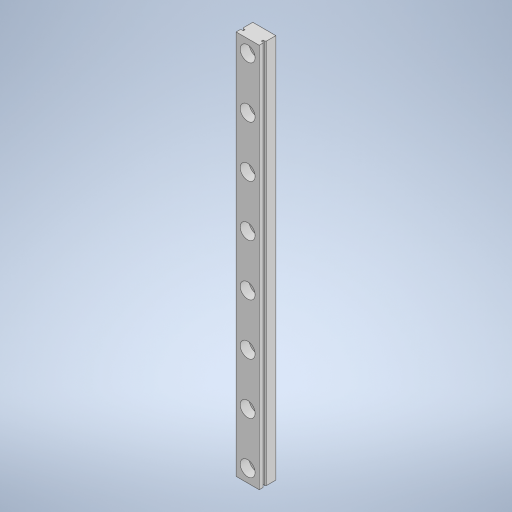
# Autodesk Inventor part: rail
Saved by Autodesk Inventor 2024 (Build 280153000, 153)
## iProperties
Created: 2025-06-01
Part Number: rail
Material: 一般
Document SubType Name: Modeling
Designer: 1412z
Density: 1 g/cm^3
Appearance: 既定
Author: 1412z
Autodesk Inventor part; units mm, degrees
ref_plane "YZ Plane" through (0, 0, 0) normal (1, 0, 0) x (0, 1, 0)
ref_plane "XZ Plane" through (0, 0, 0) normal (0, 1, 0) x (-1, 0, 0)
ref_plane "XY Plane" through (0, 0, 0) normal (0, 0, 1) x (1, 0, 0)
sketch "スケッチ1" plane through (0, 0, 0) normal (0, 0, 1) x (1, 0, 0)
  line L0 (-4.5, 75) -> (4.5, 75)
  line L1 (4.5, 75) -> (4.5, -75)
  line L2 (4.5, -75) -> (-4.5, -75)
  line L3 (-4.5, -75) -> (-4.5, 75)
  line L4 (-4.5, 75) -> (4.5, -75) construction
  line L5 (4.5, 75) -> (-4.5, -75) construction
  circle A0 centre (0, 70) radius 1.7
  circle A1 centre (0, 50) radius 1.7
  circle A2 centre (0, 30) radius 1.7
  circle A3 centre (0, 10) radius 1.7
  circle A4 centre (0, -10) radius 1.7
  circle A5 centre (0, -30) radius 1.7
  circle A6 centre (0, -50) radius 1.7
  circle A7 centre (0, -70) radius 1.7
  point P0 (0, 0)
  dimension "d0" = 9
  dimension "d1" = 150
  dimension "d2" = 3.4
  dimension "d3" = 3.4
  dimension "d4" = 3.4
  dimension "d5" = 3.4
  dimension "d6" = 3.4
  dimension "d7" = 3.4
  dimension "d8" = 3.4
  dimension "d9" = 3.4
  constraints: 12 end point, 8 centre point, 2 midpoint, 2 parallel, 1 horizontal, 1 perpendicular
  measures "d0" distance of L1.end L2.end
  measures "d1" distance of L0.end L1.end
  measures "d2" diameter of A0
  measures "d3" diameter of A1
  measures "d4" diameter of A2
  measures "d5" diameter of A3
  measures "d6" diameter of A4
  measures "d7" diameter of A5
  measures "d8" diameter of A6
  measures "d9" diameter of A7
extrude "押し出し1" add sketch "スケッチ1" along normal blind 6.5
sketch "スケッチ2" plane through (0, 0, 6.5) normal (0, 0, 1) x (1, 0, 0)
  circle A0 centre (0, -70) radius 1.7 projected
  circle A1 centre (0, -70) radius 2.9
  circle A2 centre (0, -50) radius 1.7 projected
  circle A3 centre (0, -50) radius 2.9
  circle A4 centre (0, -30) radius 1.7 projected
  circle A5 centre (0, -30) radius 2.9
  circle A6 centre (0, -10) radius 1.7 projected
  circle A7 centre (0, -10) radius 2.9
  circle A8 centre (0, 10) radius 1.7 projected
  circle A9 centre (0, 10) radius 2.9
  circle A10 centre (0, 30) radius 1.7 projected
  circle A11 centre (0, 30) radius 2.9
  circle A12 centre (0, 50) radius 1.7 projected
  circle A13 centre (0, 50) radius 2.9
  circle A14 centre (0, 70) radius 1.7 projected
  circle A15 centre (0, 70) radius 2.9
  point P0 (0, 0)
  dimension "d12" = 5.8
  dimension "d13" = 5.8
  dimension "d14" = 5.8
  dimension "d15" = 5.8
  dimension "d16" = 5.8
  dimension "d17" = 5.8
  dimension "d18" = 5.8
  dimension "d19" = 5.8
  constraints: 8 centre point, 8 coincident
  measures "d12" diameter of A1
  measures "d13" diameter of A3
  measures "d14" diameter of A5
  measures "d15" diameter of A7
  measures "d16" diameter of A9
  measures "d17" diameter of A11
  measures "d18" diameter of A13
  measures "d19" diameter of A15
extrude "押し出し2" cut sketch "スケッチ2" against normal blind 3.5
sketch "スケッチ3" plane through (-4.5, 75, 0) normal (0, 1, 0) x (1, 0, 0)
  line L0 (9, 0) -> (9, -6.5) projected
  line L1 (9, -4) -> (8, -4)
  line L2 (9, -4) -> (10, -4) construction
  line L3 (8, -4) -> (8, -4.7)
  line L4 (8, -4.7) -> (9, -4.7)
  line L5 (9, -4.7) -> (9, -4)
  line L6 (0, 0) -> (0, -6.5) projected
  line L7 (0, -4.7) -> (1, -4.7)
  line L8 (1, -4.7) -> (1, -4)
  line L9 (1, -4) -> (0, -4)
  line L10 (0, -4.7) -> (0, -4)
  point P0 (4.5, 0)
  dimension "d22" = 1
  dimension "d23" = 180
  dimension "d24" = 0.7
  dimension "d25" = 1
  constraints: 18 end point, 8 point on line, 5 perpendicular, 2 collinear, 1 horizontal
  measures "d22" distance of L1.start L1.end
  measures "d23" angle of L1 L2
  measures "d24" distance of L1.end L3.end
  measures "d25" distance of L7.start L7.end
extrude "押し出し3" cut sketch "スケッチ3" against normal blind 150
chamfer "面取り1" distance 0.3 angle 45 4 edges at (4.5, 0, 4) (4.5, 0, 4.7) (-4.5, 0, 4) (-4.5, 0, 4.7)
chamfer "面取り2" distance 0.3 angle 45 8 edges at (-1.7, 70, 0) (-1.7, 50, 0) (-1.7, 30, 0) (-1.7, 10, 0) (-1.7, -10, 0) (-1.7, -30, 0) (-1.7, -50, 0) (-1.7, -70, 0)
